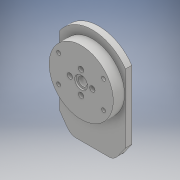
# Autodesk Inventor part: table_2
Saved by Autodesk Inventor 2018 (Build 220112000, 112)
## iProperties
Created: 2018-02-04
Part Number: table_2
Material: Generic
Document SubType Name: Modeling
Designer: Clevo
Density: 1 g/cm^3
Appearance: Default
Author: Clevo
Autodesk Inventor part; units mm, degrees
ref_plane "YZ Plane" through (0, 0, 0) normal (1, 0, 0) x (0, 1, 0)
ref_plane "XZ Plane" through (0, 0, 0) normal (0, 1, 0) x (-1, 0, 0)
ref_plane "XY Plane" through (0, 0, 0) normal (0, 0, 1) x (1, 0, 0)
sketch "Sketch1" plane through (0, 0, 0) normal (0, 1, 0) x (-1, 0, 0)
  circle A0 centre (0, 0) radius 20
  dimension "d0" = 40
  constraints: 1 centre point, 1 coincident
  measures "d0" diameter of A0
extrude "Extrusion1" add sketch "Sketch1" along normal blind 7
sketch "Sketch2" plane through (0, 7, 0) normal (0, 1, 0) x (1, 0, 0)
  circle A0 centre (0, 0) radius 40.2
  dimension "d3" = 80.4
  constraints: 1 centre point, 1 coincident
  measures "d3" diameter of A0
extrude "Extrusion2" add sketch "Sketch2" along normal blind 4
sketch "Sketch3" plane through (0, 0, 0) normal (0, -1, 0) x (1, 0, 0)
  point P0 (0, 0)
  point P1 (0, 7)
  dimension "d6" = 7
  constraints: 1 vertical alignment
  measures "d6" distance of point (0, 0) point (0, 7)
hole "Hole1" at (0, 0, 7) direction (0, 1, 0) diameter 3.3 end through all clearance for "Flat Head Machine Screw" size "M3" standard "Ansi Metric M Profile"
pattern_circular "Circular Pattern1" count 4 over 360 about axis through (0, -10, 0) along (0, 1, 0) of "Hole1"
sketch "Sketch4" plane through (0, 11, 0) normal (0, 1, 0) x (1, 0, 0)
  circle A0 centre (0, 0) radius 2.75
  dimension "d17" = 5.5
  constraints: 1 centre point, 1 coincident
  measures "d17" diameter of A0
extrude "Extrusion3" cut sketch "Sketch4" against normal up to surface (11 mm away)
sketch "Sketch5" plane through (0, 0, 0) normal (0, -1, 0) x (1, 0, 0)
  circle A0 centre (0, 0) radius 4
  dimension "d20" = 8
  constraints: 1 centre point, 1 coincident
  measures "d20" diameter of A0
extrude "Extrusion4" cut sketch "Sketch5" against normal blind 1
sketch "Sketch6" plane through (0, 11, 0) normal (0, 1, 0) x (1, 0, 0)
  circle A0 centre (0, 0) radius 2.75 projected
  circle A1 centre (-7, 0) radius 1.65 projected
  circle A2 centre (0, 7) radius 1.65 projected
  circle A3 centre (7, 0) radius 1.65 projected
  circle A4 centre (0, -7) radius 1.65 projected
  circle A5 centre (0, 0) radius 40.2 projected
  circle A6 centre (0, -7) radius 2.85
  dimension "d23" = 5.7
  constraints: 1 centre point, 1 coincident
  measures "d23" diameter of A6
extrude "Extrusion5" cut sketch "Sketch6" against normal blind 4 contours A6
pattern_circular "Circular Pattern2" count 4 over 360 about axis through (0, 11, 0) along (0, -1, 0) of "Extrusion5"
sketch "Sketch8" plane through (0, 11, 0) normal (0, 1, 0) x (1, 0, 0)
  line L0 (-14, -9) -> (14, -9)
  line L1 (14, -9) -> (14, 8)
  line L2 (14, 8) -> (-14, 8)
  line L3 (-14, 8) -> (-14, -9)
  circle A0 centre (7, 0) radius 2.85 projected
  circle A1 centre (0, 7) radius 2.85 projected
  circle A2 centre (-7, 0) radius 2.85 projected
  circle A3 centre (0, -7) radius 2.85 projected
  circle A4 centre (0, 0) radius 2.75 projected
  circle A5 centre (0, 0) radius 40.2 projected
  dimension "d29" = 17
  dimension "d30" = 28
  dimension "d31" = 7
  dimension "d32" = 7
  dimension "d33" = 2
  constraints: 8 end point, 2 parallel, 1 horizontal, 1 perpendicular
  measures "d29" distance of L2.end L0.start
  measures "d30" distance of L0.start L0.end
  measures "d31" distance from line of A0.centre L1
  measures "d32" distance from line of L3 A2.centre
  measures "d33" distance from line of L0 A3.centre
hole "Hole2" at (-14, 11, 9) at (14, 11, 9) at (14, 11, -8) at (-14, 11, -8) direction (0, -1, 0) diameter 2.459 end through all thread size "M3x0.5" class "6H" standard "ANSI Metric M Profile"
sketch "Sketch9" plane through (0, 11, 0) normal (0, 1, 0) x (1, 0, 0)
  circle A0 centre (-14, 8) radius 1.65 projected
  circle A1 centre (-14, -9) radius 1.65 projected
  arc A2 (-18.8931, -15.6569) -> (-13.2363, -18) centre (-13.2363, -10) ccw projected
  line L0 (-20.55, -14) -> (-18.8931, -15.6569) projected
  line L1 (-20.55, -14) -> (-20.55, 28.669) projected
  line L2 (-15.8931, 35.2548) -> (-20.55, 28.669) projected
  ellipse E0 centre (-10.2363, 27.2548) end of major axis (-10.2363, 38.5685) minor radius 8 (-10.2363, 38.5685) -> (-15.8931, 35.2548) ccw projected
  line L3 (-10.2363, 38.5685) -> (0, 38.5685) projected
  line L4 (0, -18) -> (0, 38.5685) projected
  line L5 (0, -18) -> (-13.2363, -18) projected
  circle A3 centre (14, 8) radius 1.65 projected
  circle A4 centre (14, -9) radius 1.65 projected
  arc A5 (13.2363, -18) -> (18.8931, -15.6569) centre (13.2363, -10) ccw projected
  line L6 (0, -18) -> (13.2363, -18) projected
  line L7 (0, 38.5685) -> (0, -18) projected
  line L8 (10.2363, 38.5685) -> (0, 38.5685) projected
  ellipse E1 centre (10.2363, 27.2548) end of major axis (10.2363, 38.5685) minor radius 8 (15.8931, 35.2548) -> (10.2363, 38.5685) ccw projected
  line L9 (20.55, 28.669) -> (15.8931, 35.2548) projected
  line L10 (20.55, 28.669) -> (20.55, -14) projected
  line L11 (18.8931, -15.6569) -> (20.55, -14) projected
  circle A6 centre (0, 0) radius 2.75 projected
  circle A7 centre (0, 0) radius 85.5095
  circle A8 centre (0, 0) radius 20 projected
  arc A9 (20.55, -14) -> (20.55, 14) centre (0, 0) ccw
  arc A10 (-20.55, -14) -> (20.55, -14) centre (0, 0) ccw
  arc A11 (20.55, 14) -> (-20.55, 14) centre (0, 0) ccw
  arc A12 (-20.55, 14) -> (-20.55, -14) centre (0, 0) ccw
  constraints: 8 point on circle, 5 centre point, 2 end point, 2 point on line, 1 coincident, 2 other
extrude "Extrusion6" cut sketch "Sketch9" against normal up to surface (11 mm away) contours A12 L1 | L10 A9 | A7
equation "\"d31\" = d32"
body "Solid1"
